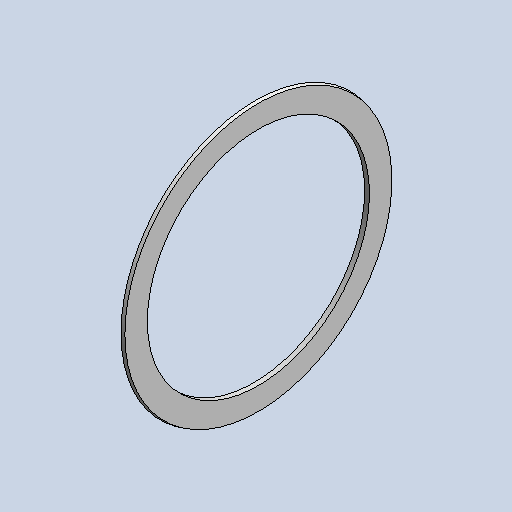
# Autodesk Inventor part: Cube
Saved by Autodesk Inventor 2025.3 (Build 293356030, 356C)
## iProperties
Shininess: 0.0
Created: 2022-05-05
Part Number: Cube
Material: PLA filament
Document SubType Name: Modeling
Mass: 7.14985 g
Surface Area: 90.3589 cm^2
Volume: 5.95821 cm^3
Density: 1.2 g/cm^3
Appearance: 일반
Density: 0.0
Volumn: 0.0
Area: 0.0
PropertySet Name: Model Information
Control State: 0
Master: False
Checked Out: False
Author: Administrateur
Autodesk Inventor part; units mm, degrees
ref_plane "YZ Plane" through (0, 0, 0) normal (1, 0, 0) x (0, 1, 0)
ref_plane "XZ Plane" through (0, 0, 0) normal (0, 1, 0) x (-1, 0, 0)
ref_plane "XY Plane" through (0, 0, 0) normal (0, 0, 1) x (1, 0, 0)
sketch "스케치1" plane through (0, 0, 0) normal (0, 0, 1) x (1, 0, 0)
  line L0 (2.2715, 63.1118) -> (2.2715, -63.1118) projected
  line L1 (0, 60.43) -> (0, -60.43) projected
  line L2 (0, 60.43) -> (0.8226, 63.5) projected
  line L3 (2.2715, 63.1118) -> (0.8226, 63.5) projected
  line L4 (0, 0) -> (8.4353, 0)
  point P0 (2.2715, 0)
  constraints: 2 end point, 1 horizontal
revolve "회전1" add sketch "스케치1" angle 360 about axis through (0, 0, 0) along (1, 0, 0)
sketch "스케치2" plane through (2.2715, 0, 0) normal (1, 0, 0) x (0, 0, -1)
  circle A0 centre (0, 0) radius 52.5
  dimension "d1" = 105
  constraints: 1 centre point, 1 coincident
  measures "d1" diameter of A0
extrude "돌출1" cut sketch "스케치2" against normal through all
equation "\"joint4_belt_centor\" = 157.367"
equation "\"joint4_axis2_L\" = 58.803"
equation "\"joint4_axis2_b1\" = 35"
equation "\"joint4_axis2_d\" = 19"
equation "\"joint4_miter_m\" = 2"
equation "\"joint4_miter_a\" = 20deg"
equation "\"joint4_miter_z\" = 79"
equation "\"joint4_miter_b\" = 6.90139"
equation "\"joint4_axis3_L\" = 23.5"
equation "\"joint3_belt_centor\" = 157.367"
equation "\"joint3_axis2_L\" = 63.75"
equation "\"joint3_axis2_b1\" = 38"
equation "\"joint3_axis2_d\" = 29"
equation "\"joint3_planetary_m\" = 2"
equation "\"joint3_planetary_a\" = 20deg"
equation "\"joint3_planetary_np\" = 4"
equation "\"joint3_sun_b\" = 19"
equation "\"joint3_planet_b\" = 19"
equation "\"joint3_ring_b\" = 18"
equation "\"joint3_axis3_d\" = 29"
equation "\"joint3_miter_m\" = 4"
equation "\"joint3_miter_a\" = 20deg"
equation "\"joint3_miter_z\" = 28"
equation "\"joint3_miter_b\" = 25.07657"
equation "\"joint3_axis4_L\" = 43.706"
equation "\"joint3_miter_z2\" = 39"
equation "\"joint3_miter_z1\" = 26"
